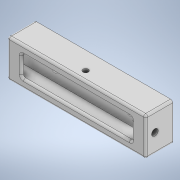
# Autodesk Inventor part: Part1
Saved by Autodesk Inventor 2021.4 (Build 254397000, 397)
## iProperties
Created: 2023-11-13
Part Number: Part1
Material: 一般
Document SubType Name: Modeling
Designer: ryusei
Density: 1 g/cm^3
Appearance: 既定
Author: ryusei
Autodesk Inventor part; units mm, degrees
ref_plane "YZ Plane" through (0, 0, 0) normal (1, 0, 0) x (0, 1, 0)
ref_plane "XZ Plane" through (0, 0, 0) normal (0, 1, 0) x (-1, 0, 0)
ref_plane "XY Plane" through (0, 0, 0) normal (0, 0, 1) x (1, 0, 0)
sketch "スケッチ1" plane through (0, 0, 0) normal (0, 0, 1) x (1, 0, 0)
  line L0 (-64, 17.5) -> (64, 17.5)
  line L1 (64, 17.5) -> (64, -17.5)
  line L2 (64, -17.5) -> (-64, -17.5)
  line L3 (-64, -17.5) -> (-64, 17.5)
  line L4 (-64, 17.5) -> (64, -17.5) construction
  line L5 (64, 17.5) -> (-64, -17.5) construction
  point P0 (0, 0)
  dimension "d0" = 128
  dimension "d1" = 35
  constraints: 12 end point, 2 midpoint, 2 parallel, 1 horizontal, 1 perpendicular
  measures "d0" distance of L1.end L2.end
  measures "d1" distance of L0.end L1.end
extrude "押し出し1" add sketch "スケッチ1" along normal blind 25
sketch "スケッチ3" plane through (-64, -17.5, 0) normal (-1, 0, 0) x (0, 0, 1)
  line L0 (10, 30) -> (23, 30)
  line L1 (23, 30) -> (23, 5)
  line L2 (23, 5) -> (10, 5)
  line L3 (10, 5) -> (10, 30)
  line L4 (0, 0) -> (25, 0) projected
  line L5 (25, 35) -> (25, 0) projected
  point P0 (0, 17.5)
  dimension "d8" = 13
  dimension "d9" = 25
  dimension "d10" = 5
  dimension "d11" = 2
  constraints: 8 end point, 2 parallel, 1 horizontal, 1 perpendicular
  measures "d8" distance of L1.end L2.end
  measures "d9" distance of L0.end L1.end
  measures "d10" distance between parallel lines of L4 L2
  measures "d11" distance between parallel lines of L5 L1
extrude "押し出し2" cut sketch "スケッチ3" against normal blind 118
sketch "スケッチ4" plane through (0, 0, 25) normal (0, 0, 1) x (1, 0, 0)
  line L0 (-51, 9.5) -> (51, 9.5)
  line L1 (51, 9.5) -> (51, -9.5)
  line L2 (51, -9.5) -> (-51, -9.5)
  line L3 (-51, -9.5) -> (-51, 9.5)
  line L4 (-51, 9.5) -> (51, -9.5) construction
  line L5 (51, 9.5) -> (-51, -9.5) construction
  point P0 (0, 0)
  dimension "d14" = 102
  dimension "d15" = 19
  constraints: 12 end point, 2 midpoint, 2 parallel, 1 horizontal, 1 perpendicular
  measures "d14" distance of L0.start L0.end
  measures "d15" distance of L0.end L1.end
extrude "押し出し3" cut sketch "スケッチ4" against normal blind 2
sketch "スケッチ6" plane through (64, -17.5, 0) normal (1, 0, 0) x (0, 0, -1)
  line L0 (0, 0) -> (-25, 0) projected
  line L1 (0, 0) -> (0, 35) projected
  line L2 (-25, 0) -> (-25, 35) projected
  point P0 (0, 17.5)
  point P1 (-16.5, 17.5)
  dimension "d27" = 17.5
  dimension "d46" = 8.5
  measures "d27" distance from line of L0 point (-16.5, 17.5)
  measures "d46" distance from line of L2 point (-16.5, 17.5)
hole "穴2" at (64, 0, 16.5) direction (-1, 0, 0) diameter 6 end through all
sketch "スケッチ7" plane through (-64, 17.5, 0) normal (0, 1, 0) x (1, 0, 0)
  line L0 (128, 0) -> (0, 0) projected
  line L1 (128, 0) -> (128, -25) projected
  line L2 (128, -25) -> (0, -25) projected
  point P0 (64, 0)
  point P1 (64, -16.5)
  dimension "d37" = 64
  dimension "d45" = 8.5
  measures "d37" distance from line of L1 point (64, -16.5)
  measures "d45" distance from line of L2 point (64, -16.5)
hole "穴3" at (0, 17.5, 16.5) direction (0, -1, 0) diameter 4.9 depth 8
sketch "スケッチ8" plane through (-64, -12.5, 10) normal (0, 0, 1) x (1, 0, 0)
  point P0 (64, 12.5)
  point P1 (29, 12.5)
  point P2 (99, 12.5)
  dimension "d47" = 35
  dimension "d48" = 35
  measures "d47" distance of point (29, 12.5) point (64, 12.5)
  measures "d48" distance of point (99, 12.5) point (64, 12.5)
hole "穴4" at (-35, 0, 10) at (35, 0, 10) direction (0, 0, -1) diameter 6 depth 15 counterbore diameter 10 counterbore depth 6
fillet "フィレット1" radius 2 12 edges at (-64, 17.5, 12.5) (0, 17.5, 25) (0, -17.5, 25) (-64, -17.5, 12.5) (64, 17.5, 12.5) (-64, 0, 25) (64, 0, 25) (64, -17.5, 12.5) (-51, 9.5, 24) (-51, -9.5, 24) (51, -9.5, 24) (51, 9.5, 24)
fillet "フィレット2" radius 2 8 edges at (50.4142, 8.9142, 25) (51, 0, 25) (50.4142, -8.9142, 25) (0, -9.5, 25) (-50.4142, -8.9142, 25) (-51, 0, 25) (-50.4142, 8.9142, 25) (0, 9.5, 25)
